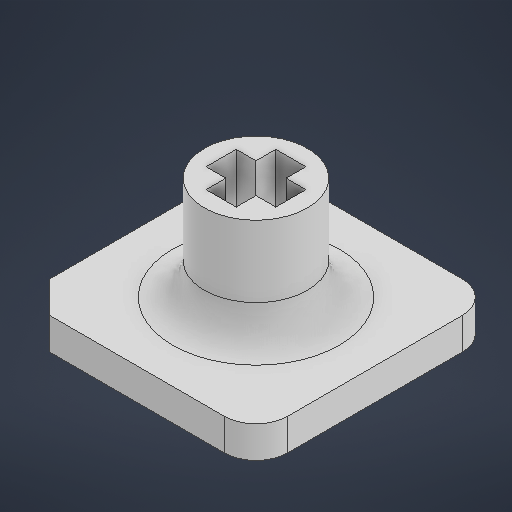
# Autodesk Inventor part: button_3d
Saved by Autodesk Inventor 2026 (Build 300175000, 175)
## iProperties
Created: 2025-05-11
Part Number: button_3d
Material: 일반
Document SubType Name: Modeling
Designer: encle
Density: 1 g/cm^3
Appearance: 기본값
Author: encle
Autodesk Inventor part; units mm, degrees
ref_plane "YZ Plane" through (0, 0, 0) normal (1, 0, 0) x (0, 1, 0)
ref_plane "XZ Plane" through (0, 0, 0) normal (0, 1, 0) x (-1, 0, 0)
ref_plane "XY Plane" through (0, 0, 0) normal (0, 0, 1) x (1, 0, 0)
sketch "스케치1" plane through (0, 0, 0) normal (0, 1, 0) x (-1, 0, 0)
  line L0 (2.2, -0.95) -> (-2.2, -0.95)
  line L1 (-2.2, -0.95) -> (-2.2, 0.95)
  line L2 (-2.2, 0.95) -> (2.2, 0.95)
  line L3 (2.2, 0.95) -> (2.2, -0.95)
  line L4 (2.2, -0.95) -> (-2.2, 0.95) construction
  line L5 (-2.2, -0.95) -> (2.2, 0.95) construction
  point P0 (0, 0)
  dimension "d0" = 4.4
  dimension "d1" = 1.9
  constraints: 12 end point, 2 midpoint, 2 parallel, 1 horizontal, 1 perpendicular
  measures "d0" distance of L1.end L2.end
  measures "d1" distance of L0.end L1.end
sketch "스케치2" plane through (0, 0, 0) normal (0, 1, 0) x (-1, 0, 0)
  line L0 (-0.95, -2.2) -> (0.95, -2.2)
  line L1 (0.95, -2.2) -> (0.95, 2.2)
  line L2 (0.95, 2.2) -> (-0.95, 2.2)
  line L3 (-0.95, 2.2) -> (-0.95, -2.2)
  line L4 (-0.95, -2.2) -> (0.95, 2.2) construction
  line L5 (0.95, -2.2) -> (-0.95, 2.2) construction
  point P0 (0, 0)
  dimension "d2" = 1.9
  dimension "d3" = 4.4
  constraints: 12 end point, 2 midpoint, 2 parallel, 1 horizontal, 1 perpendicular
  measures "d2" distance of L2.end L1.end
  measures "d3" distance of L1.end L0.end
sketch "스케치3" plane through (0, 0, 0) normal (0, 1, 0) x (-1, 0, 0)
  circle A0 centre (0, 0) radius 3.25
  line L0 (-0.95, 2.2) -> (-0.95, -2.2) projected
  line L1 (0.95, 2.2) -> (-0.95, 2.2) projected
  line L2 (0.95, -2.2) -> (0.95, 2.2) projected
  line L3 (2.2, -0.95) -> (-2.2, -0.95) projected
  line L4 (-2.2, -0.95) -> (-2.2, 0.95) projected
  line L5 (-2.2, 0.95) -> (2.2, 0.95) projected
  line L6 (2.2, 0.95) -> (2.2, -0.95) projected
  line L7 (2.2, -0.95) -> (-2.2, 0.95) construction
  line L8 (-2.2, -0.95) -> (2.2, 0.95) construction
  line L9 (-0.95, -2.2) -> (0.95, -2.2) projected
  line L10 (-0.95, -2.2) -> (0.95, 2.2) construction
  line L11 (0.95, -2.2) -> (-0.95, 2.2) construction
  point P0 (0.95, 0.95)
  point P1 (0.95, -0.95)
  point P2 (-0.95, -0.95)
  point P3 (-0.95, 0.95)
  dimension "d4" = 6.5
  constraints: 1 centre point, 1 coincident
  measures "d4" diameter of A0
extrude "돌출1" add sketch "스케치3" along normal blind 6.5
sketch "스케치4" plane through (0, 0, 0) normal (0, -1, 0) x (1, 0, 0)
  line L0 (7.5, 7.5) -> (-7.5, 7.5)
  line L1 (-7.5, 7.5) -> (-7.5, -7.5)
  line L2 (-7.5, -7.5) -> (7.5, -7.5)
  line L3 (7.5, -7.5) -> (7.5, 7.5)
  line L4 (7.5, 7.5) -> (-7.5, -7.5) construction
  line L5 (-7.5, 7.5) -> (7.5, -7.5) construction
  point P0 (0, 0)
  dimension "d7" = 15
  dimension "d8" = 15
  constraints: 12 end point, 2 midpoint, 2 parallel, 1 horizontal, 1 perpendicular
  measures "d7" distance of L2.end L1.end
  measures "d8" distance of L1.end L0.end
extrude "돌출2" add sketch "스케치4" along normal blind 2
fillet "모깎기1" radius 2 1 edges at (3.25, 0, 0)
fillet "모깎기2" radius 2 3 edges at (7.5, -1, 7.5) (7.5, -1, -7.5) (-7.5, -1, -7.5)
chamfer "모따기1" distance 2 angle 45 1 edges at (-7.5, -1, 7.5)
